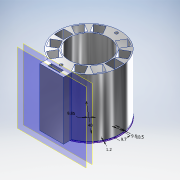
# Autodesk Inventor part: StatorShell MH
Saved by Autodesk Inventor 2018 (Build 220112000, 112)
## iProperties
Created: 2018-01-24
Part Number: StatorShell MH
Material: Aluminum 6061
Document SubType Name: Modeling
Designer: Moochster
Density: 2.7 g/cm^3
Appearance: Aluminum - Flat
Author: Moochster
Autodesk Inventor part; units mm, degrees
ref_plane "YZ Plane" through (0, 0, 0) normal (1, 0, 0) x (0, 1, 0)
ref_plane "XY Plane" through (0, 0, 0) normal (0, 0, 1) x (1, 0, 0)
sketch "Sketch1" plane through (0, 0, 0) normal (0, 0, 1) x (1, 0, 0)
  circle A0 centre (0, 0) radius 20
  circle A1 centre (0, 0) radius 30.5
  line L0 (20.9, 4.85) -> (30.5, 4.85)
  line L1 (30.5, 4.85) -> (30.5, -4.85)
  line L2 (30.5, -4.85) -> (20.9, -4.85)
  line L3 (20.9, -4.85) -> (20.9, 4.85)
  circle A2 centre (0, 0) radius 4.925
  circle A3 centre (0, 0) radius 31.7
  point P0 (20.9, 0)
  dimension "d0" = 40
  dimension "d1" = 10.5
  dimension "d2" = 9.6
  dimension "d3" = 9.7
  dimension "d11" = 9.85
  dimension "d14" = 1.2
  constraints: 8 end point, 4 centre point, 4 coincident, 2 parallel, 1 horizontal, 1 horizontal alignment, 1 midpoint, 1 perpendicular, 1 tangent
  measures "d0" diameter of A0
  measures "d1" radial gap between concentric circles of A0 A1
  measures "d2" distance of L0.start L0.end
  measures "d3" distance of L0.end L1.end
  measures "d11" diameter of A2
  measures "d14" radial gap between concentric circles of A1 A3
extrude "Extrusion1" add sketch "Sketch1" along normal blind 60 contours A1 L2 L3 L0 | L0 L3 L2 A1
extrude "Extrusion2" add sketch "Sketch1" against normal blind 5 contours A0 | A1 L2 L3 L0 | L0 L3 L2 A1
extrude "Extrusion3" cut sketch "Sketch1" along normal through all both and the other way through all contours A1 L2 L3 L0 | L1 L2 A1 | A1 L0 L1 picked at (24.1, 0)
pattern_circular "Circular Pattern1" count 3 over 60 about axis through (0, 0, 0) along (0, 0, 1) of "Extrusion3"
mirror "Mirror1" about plane through (0, 0, 0) normal (0, 1, 0) of "Extrusion3", "Circular Pattern1"
mirror "Mirror2" about plane through (0, 0, 0) normal (1, 0, 0) of "Extrusion3", "Circular Pattern1", "Mirror1"
extrude "Extrusion4" add sketch "Sketch1" along normal up to surface (60 mm away) contours A3
chamfer "Chamfer1" distance 5 angle 45 10 edges at (21.5668, 21.5668, -5) (29.4607, 7.894, -5) (29.4607, -7.894, -5) (21.5668, -21.5668, -5) (0, -30.5, -5) (0, 30.5, -5) (-21.5668, 21.5668, -5) (-29.4607, 7.894, -5) (-29.4607, -7.894, -5) (-21.5668, -21.5668, -5)
chamfer "Chamfer2" distance 1.2 angle 45 1 edges at (-31.7, 0, 0)
sketch "Sketch2" plane through (0, 0, 60) normal (0, 0, 1) x (1, 0, 0)
  point P0 (0, 0)
  point P1 (0, -28)
  point P2 (0, 28)
  dimension "d20" = 56
  dimension "d21" = 28
  constraints: 2 vertical alignment
  measures "d20" distance of point (0, -28) point (0, 28)
  measures "d21" distance of point (0, 0) point (0, -28)
hole "Hole1" at (0, -28, 60) at (0, 28, 60) direction (0, 0, -1) diameter 3 depth 8 tip angle 118
ref_plane "Work Plane2" through (0, -37.7, 0) normal (0, 1, 0) x (-1, 0, 0)
ref_plane "Work Plane1" through (0, -31.7, 0) normal (0, 1, 0) x (-1, 0, 0)
sketch "Sketch3" plane through (0, -37.7, 0) normal (0, 1, 0) x (-1, 0, 0)
  line L0 (-12, 60) -> (12, 60)
  line L1 (12, 60) -> (12, 1.2)
  line L2 (12, 1.2) -> (-12, 1.2)
  line L3 (-12, 1.2) -> (-12, 60)
  line L4 (-10.8557, 60) -> (-6.2498, 60) projected
  line L5 (-31.7, 1.2) -> (31.7, 1.2) projected
  point P0 (0, 0)
  point P1 (0, 60)
  dimension "d33" = 24
  constraints: 8 end point, 2 parallel, 1 collinear, 1 horizontal, 1 midpoint, 1 perpendicular, 1 point on line, 1 vertical alignment
  measures "d33" distance between parallel lines of L1 L3
extrude "Extrusion5" add sketch "Sketch3" along normal up to next
sketch "Sketch4" plane through (0, 0, 60) normal (0, 0, 1) x (1, 0, 0)
  line L0 (-6, -35.7) -> (6, -35.7)
  line L1 (6, -35.7) -> (6, -31.7)
  line L2 (6, -31.7) -> (-6, -31.7)
  line L3 (-6, -31.7) -> (-6, -35.7)
  line L4 (-44.38, -37.7) -> (44.38, -37.7) projected
  line L5 (12, -37.7) -> (-12, -37.7) projected
  point P0 (0, 0)
  point P1 (0, -31.7)
  point P2 (0, -37.7)
  dimension "d36" = 2
  dimension "d37" = 4
  dimension "d38" = 12
  constraints: 8 end point, 2 midpoint, 2 parallel, 1 horizontal, 1 perpendicular, 1 vertical alignment
  measures "d36" distance between parallel lines of L4 L0
  measures "d37" distance of L0.end L1.end
  measures "d38" distance of L0.start L0.end
extrude "Extrusion6" cut sketch "Sketch4" against normal blind 8
body "Solid1"
